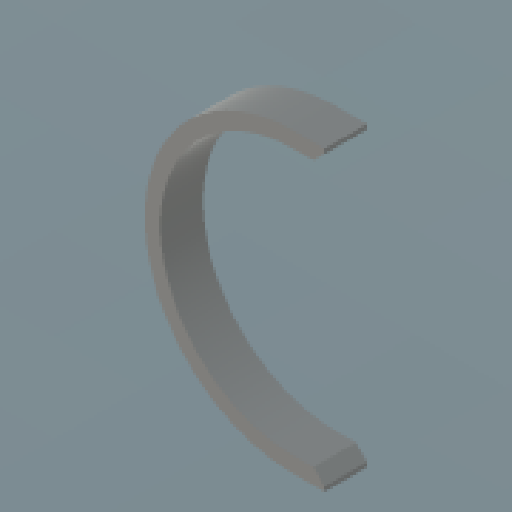
# Autodesk Inventor part: Z Drag Chain Dummy
Saved by Autodesk Inventor 2023.2 (Build 272271000, 271)
## iProperties
Created: 2023-02-19
Part Number: Z Drag Chain Dummy
Material: ABS Plastic
Document SubType Name: Modeling
Designer: remop
Density: 1.06 g/cm^3
Appearance: Gray
Author: remop
Autodesk Inventor part; units mm, degrees
ref_plane "YZ Plane" through (0, 0, 0) normal (1, 0, 0) x (0, 1, 0)
ref_plane "XZ Plane" through (0, 0, 0) normal (0, 1, 0) x (-1, 0, 0)
ref_plane "XY Plane" through (0, 0, 0) normal (0, 0, 1) x (1, 0, 0)
sketch "Sketch1" plane through (0, 0, 0) normal (0, 0, 1) x (1, 0, 0)
  line L0 (0, -10) -> (-28.4554, -10) projected
  line L1 (-28.4554, 0) -> (-28.4554, -10) projected
  line L2 (-28.4554, 0) -> (0, 0) projected
  line L3 (-28.4554, -24) -> (0, -24)
  line L4 (0, -24) -> (0, -10)
  line L5 (-300.8173, -290) -> (59.1827, -290) projected
  line L6 (-8.4554, -290) -> (-8.4554, -276)
  line L7 (-8.4554, -276) -> (-28.4554, -276)
  arc A0 (-28.4554, -24) -> (-28.4554, -276) centre (-28.4554, -150) ccw
  arc A1 (-28.4554, -10) -> (-28.4554, -290) centre (-28.4554, -150) ccw
  dimension "d0" = 14
  dimension "d7" = 20
  constraints: 8 end point, 4 point on circle, 3 point on line, 3 tangent, 2 centre point, 2 perpendicular, 2 vertical alignment, 1 coincident, 1 horizontal, 1 parallel, 1 vertical
  measures "d0" distance of L3.end L4.end
  measures "d7" distance of L6.end L7.end
extrude "Extrusion1" add sketch "Sketch1" against normal blind 38
chamfer "Chamfer1" distance 10 angle 45 2 edges at (0, -24, -19) (-8.4554, -290, -19)
body "Solid1"
